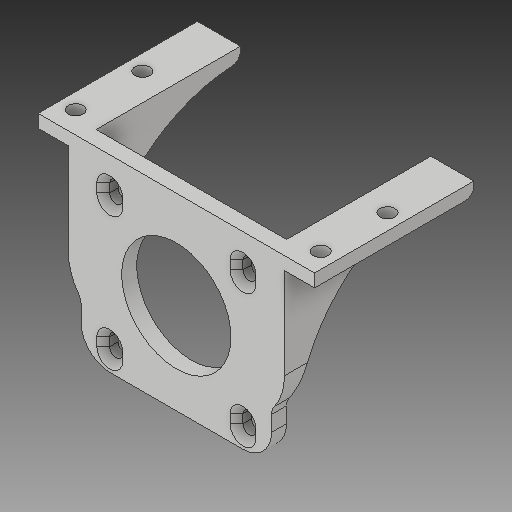
# Autodesk Inventor part: stepper mount
Saved by Autodesk Inventor 2017 (Build 210142000, 142)
## iProperties
Created: 2018-11-26
Part Number: stepper mount
Material: Generic
Document SubType Name: Modeling
Designer: Eric the Great
Density: 1 g/cm^3
Appearance: Default
Author: Eric the Great
Autodesk Inventor part; units mm, degrees
ref_plane "YZ Plane" through (0, 0, 0) normal (1, 0, 0) x (0, 1, 0)
ref_plane "XZ Plane" through (0, 0, 0) normal (0, 1, 0) x (-1, 0, 0)
ref_plane "XY Plane" through (0, 0, 0) normal (0, 0, 1) x (1, 0, 0)
sketch "Sketch1" plane through (0, 0, 0) normal (0, 0, 1) x (1, 0, 0)
  circle A0 centre (-15.5, -15.5) radius 1.5 projected
  circle A1 centre (15.5, 15.5) radius 1.5 projected
  circle A2 centre (15.5, -15.5) radius 1.5 projected
  circle A3 centre (-15.5, 15.5) radius 1.5 projected
  line L0 (21.15, 15.4142) -> (15.4142, 21.15) projected
  line L1 (15.4142, 21.15) -> (-15.4142, 21.15) projected
  line L2 (-21.15, 15.4142) -> (-15.4142, 21.15) projected
  line L3 (-21.15, 15.4142) -> (-21.15, -15.4142) projected
  line L4 (-21.15, -15.4142) -> (-15.4142, -21.15) projected
  line L5 (-15.4142, -21.15) -> (15.4142, -21.15) projected
  line L6 (21.15, -15.4142) -> (15.4142, -21.15) projected
  line L7 (21.15, -15.4142) -> (21.15, 15.4142) projected
  circle A4 centre (0, 0) radius 11 projected
  line L8 (22.15, 22.6799) -> (22.15, -14.4142)
  line L9 (15.4142, -21.15) -> (22.15, -14.4142)
  line L10 (-22.15, 22.6799) -> (-22.15, -14.4142)
  line L11 (-22.15, -14.4142) -> (-15.4142, -21.15)
  line L12 (0, 0) -> (0, -1.5411)
  line L13 (25, 22.6799) -> (-25, 22.6799) projected
  circle A5 centre (0, 0) radius 12.7
  arc A6 (15.4142, -21.15) -> (22.15, -14.4142) centre (15.4142, -14.4142) ccw
  arc A7 (-22.15, -14.4142) -> (-15.4142, -21.15) centre (-15.4142, -14.4142) ccw
  point P0 (0, 0)
  point P1 (0, 17)
  point P2 (22.15, 21.15)
  point P3 (-22.15, 21.15)
  dimension "d4" = 1
  dimension "d24" = 25.4
  constraints: 10 end point, 7 point on line, 4 point on circle, 4 tangent, 3 centre point, 2 collinear, 2 vertical, 1 coincident, 1 parallel, 1 other
  measures "d4" distance between parallel lines of L7 L8
  measures "d24" diameter of A5
extrude "Extrusion1" add sketch "Sketch1" along normal blind 3.5 contours L7 L6 L5 L4 L3 L2 L1 L0 | L0 L1 L2 L3 L11 L10 L13 L8 L9 L7 | L9 A6 L6 | A7 L11 L4
sketch "Sketch3" plane through (-22.15, -14.4142, 0) normal (-1, 0, 0) x (0, 0, 1)
  line L0 (-80.2095, 37.0941) -> (300.7905, 37.0941) projected
  line L1 (3.5, 37.0941) -> (3.5, 0) projected
  line L2 (3.5, 6.7772) -> (3.5, 37.0941)
  line L3 (-33.5642, 37.0941) -> (3.5, 37.0941)
  line L4 (0, 37.0941) -> (0, 0) projected
  arc A0 (0, 6.7772) -> (-32.2994, 34.0941) centre (-33.4606, -0.0326) ccw
  line L5 (-33.5642, 37.0941) -> (-33.5642, 34.0941)
  line L6 (-33.5642, 34.0941) -> (-32.2994, 34.0941)
  line L7 (3.5, 6.7772) -> (0, 6.7772)
  line L8 (-33.5642, 37.0941) -> (3.5, 37.0941)
  line L9 (3.5, 37.0941) -> (3.5, 33.5312)
  line L10 (-33.5642, 37.0941) -> (3.5, 37.0941)
  line L11 (3.5, 37.0941) -> (3.5, 33.5312)
  point P0 (0, 14.4142)
  point P1 (3, 35.5642)
  point P2 (0, 35.5642)
  dimension "d14" = 3
  constraints: 18 end point, 4 perpendicular, 4 point on line, 2 horizontal, 2 point on circle, 1 centre point, 1 collinear, 1 parallel, 1 vertical, 2 other
  measures "d14" distance of L3.start L5.end
extrude "Extrusion3" add sketch "Sketch3" along normal blind 3
sketch "Sketch4" plane through (22.15, -14.4142, 0) normal (1, 0, 0) x (0, 0, -1)
  arc A0 (32.2994, 34.0941) -> (0, 6.7772) centre (33.4606, -0.0326) ccw projected
  line L0 (33.5642, 34.0941) -> (32.2994, 34.0941) projected
  line L1 (33.5642, 37.0941) -> (33.5642, 34.0941) projected
  line L2 (-3.5, 6.7772) -> (0, 6.7772) projected
  line L3 (-3, 35.5642) -> (-3, 37.0941) projected
  line L4 (0, 37.0941) -> (0, 6.7772) projected
  arc A1 (32.2994, 34.0941) -> (0, 6.7772) centre (33.4606, -0.0326) ccw projected
  line L5 (33.5642, 34.0941) -> (32.2994, 34.0941) projected
  line L6 (33.5642, 37.0941) -> (33.5642, 34.0941) projected
  line L7 (0, 37.0941) -> (33.5642, 37.0941) projected
  line L8 (-3.5, 0) -> (-3.5, 37.0941) projected
  line L9 (0, 6.7772) -> (-3.5, 6.7772)
  line L10 (-3.5, 6.7772) -> (-3.5, 37.0941)
  line L11 (0, 6.7772) -> (-3.5, 6.7772)
  line L12 (-3.5, 6.7772) -> (-3.5, 37.0941)
  line L13 (-3.5, 37.0941) -> (0, 37.0941)
  line L14 (0, 37.0941) -> (0, 6.7772)
  point P0 (0, 14.4142)
  constraints: 12 end point, 2 parallel, 1 collinear, 1 horizontal, 1 perpendicular, 1 vertical, 1 other
extrude "Extrusion4" add sketch "Sketch4" along normal blind 3
sketch "Sketch5" plane through (-25.15, -14.4142, 0) normal (-1, 0, 0) x (0, 0, 1)
  line L0 (-33.5642, 37.0941) -> (3.5, 37.0941) projected
  line L1 (3.5, 37.0941) -> (3.5, 6.7772) projected
  line L2 (-33.5642, 37.0941) -> (3.5, 37.0941)
  line L3 (3.5, 37.0941) -> (3.5, 34.0941)
  line L4 (3.5, 34.0941) -> (-33.5642, 34.0941)
  line L5 (-33.5642, 34.0941) -> (-33.5642, 37.0941)
  point P0 (0, 14.4142)
  dimension "d9" = 3
  constraints: 8 end point, 2 parallel, 1 horizontal, 1 perpendicular, 1 point on line
  measures "d9" distance of L4.end L0.start
extrude "Extrusion5" add sketch "Sketch5" along normal blind 7
fillet "Fillet1" radius 3.175 2 edges at (-22.15, -7.6371, 1.75) (22.15, -7.6371, 1.75)
fillet "Fillet2" radius 12.7 4 edges at (25.15, -7.6395, 0) (25.15, -7.6419, 1.75) (-25.15, -7.6395, 0) (-25.15, -7.6419, 1.75)
sketch "Sketch6" plane through (25.15, -14.4142, 0) normal (1, 0, 0) x (0, 0, -1)
  line L0 (33.5642, 37.0941) -> (33.5642, 34.0941) projected
  line L1 (33.5642, 37.0941) -> (-3.5, 37.0941)
  line L2 (-3.5, 37.0941) -> (-3.5, 34.0941)
  line L3 (-3.5, 34.0941) -> (33.5642, 34.0941)
  line L4 (33.5642, 34.0941) -> (33.5642, 37.0941)
  line L5 (-3.5, 37.0941) -> (-3.5, 12.8941) projected
  point P0 (0, 14.4142)
  dimension "d15" = 3
  constraints: 8 end point, 2 parallel, 1 horizontal, 1 perpendicular, 1 point on line
  measures "d15" distance of L0.start L0.end
extrude "Extrusion6" add sketch "Sketch6" along normal blind 7
sketch "Sketch7" plane through (22.15, 19.6799, -33.5642) normal (0, -1, 0) x (1, 0, 0)
  circle A0 centre (6.35, 15.9631) radius 1.75 projected
  circle A1 centre (-50.65, 15.9631) radius 1.75 projected
  circle A2 centre (6.35, 31.9823) radius 1.75
  circle A3 centre (-50.65, 31.9823) radius 1.75
  circle A4 centre (6.35, 16.4631) radius 1.75 projected
  circle A5 centre (-50.65, 16.4631) radius 1.75 projected
  point P0 (-22.15, 33.5642)
  dimension "d18" = 3.5
  dimension "d19" = 3.5
  constraints: 2 centre point
  measures "d18" diameter of A2
  measures "d19" diameter of A3
extrude "Extrusion7" cut sketch "Sketch7" against normal up to surface (3 mm away) contours A4 A0 | A0 A4 | A5 A1 | A1 A5 | A2 | A3 picked at (6.4875, 16.6967) picked at (6.5821, 17.8556) picked at (-50.7875, 16.6967) picked at (-50.4179, 17.8556)
fillet "Fillet3" radius 2 2 edges at (27.15, 19.6799, -33.5642) (-27.15, 19.6799, -33.5642)
fillet "Fillet4" radius 2 2 edges at (23.65, 19.6995, -33.5642) (-23.65, 19.6995, -33.5642)
sketch "Sketch8" plane through (0, 0, 3.5) normal (0, 0, 1) x (1, 0, 0)
  arc A0 (-25.15, -1.5201) -> (-22.75, -8.9498) centre (-12.45, -1.5201) ccw projected
  arc A1 (-22.15, -10.8072) -> (-22.75, -8.9498) centre (-25.325, -10.8072) ccw projected
  line L0 (-22.15, -10.8072) -> (-22.15, -14.4142) projected
  line L1 (-15.4142, -21.15) -> (15.4142, -21.15) projected
  line L2 (22.15, -14.4142) -> (22.15, -10.8072) projected
  arc A2 (22.75, -8.9498) -> (22.15, -10.8072) centre (25.325, -10.8072) ccw projected
  arc A3 (22.75, -8.9498) -> (25.15, -1.5201) centre (12.45, -1.5201) ccw projected
  line L3 (25.15, 19.6799) -> (25.15, -1.5201) projected
  line L4 (25.15, 19.6799) -> (32.15, 19.6799) projected
  line L5 (32.15, 22.6799) -> (32.15, 19.6799) projected
  line L6 (-32.15, 22.6799) -> (32.15, 22.6799) projected
  line L7 (-32.15, 19.6799) -> (-32.15, 22.6799) projected
  line L8 (-25.15, 19.6799) -> (-32.15, 19.6799) projected
  line L9 (-25.15, -1.5201) -> (-25.15, 19.6799) projected
  circle A4 centre (-15.5, -15.5) radius 1.5 projected
  circle A5 centre (15.5, 15.5) radius 1.5 projected
  circle A6 centre (15.5, -15.5) radius 1.5 projected
  circle A7 centre (-15.5, 15.5) radius 1.5 projected
  circle A8 centre (0, 0) radius 12.7 projected
  line L10 (-15.5, 15.5) -> (-15.5, 13.5) construction
  line L11 (-17, 15.5) -> (-17, 13.5)
  line L12 (-14, 13.5) -> (-14, 15.5)
  arc A9 (-14, 15.5) -> (-17, 15.5) centre (-15.5, 15.5) ccw
  arc A10 (-17, 13.5) -> (-14, 13.5) centre (-15.5, 13.5) ccw
  line L13 (15.5, 15.5) -> (15.5, 13.5) construction
  line L14 (14, 15.5) -> (14, 13.5)
  line L15 (17, 13.5) -> (17, 15.5)
  arc A11 (17, 15.5) -> (14, 15.5) centre (15.5, 15.5) ccw
  arc A12 (14, 13.5) -> (17, 13.5) centre (15.5, 13.5) ccw
  line L16 (-15.5, -15.5) -> (-15.5, -17.5) construction
  line L17 (-14, -15.5) -> (-14, -17.5)
  line L18 (-17, -17.5) -> (-17, -15.5)
  arc A13 (-14, -15.5) -> (-17, -15.5) centre (-15.5, -15.5) ccw
  arc A14 (-17, -17.5) -> (-14, -17.5) centre (-15.5, -17.5) ccw
  circle A15 centre (15.5, -15.5) radius 1.5 projected
  line L19 (15.5, -15.5) -> (15.5, -17.5) construction
  line L20 (14, -15.5) -> (14, -17.5)
  line L21 (17, -17.5) -> (17, -15.5)
  arc A16 (17, -15.5) -> (14, -15.5) centre (15.5, -15.5) ccw
  arc A17 (14, -17.5) -> (17, -17.5) centre (15.5, -17.5) ccw
  arc A18 (-22.15, -14.4142) -> (-15.4142, -21.15) centre (-15.4142, -14.4142) ccw projected
  arc A19 (15.4142, -21.15) -> (22.15, -14.4142) centre (15.4142, -14.4142) ccw projected
  circle A20 centre (-15.5, -15.5) radius 1.5 projected
  point P0 (0, 0)
  point P1 (-15.5, 14.5)
  point P2 (15.5, 14.5)
  point P3 (-15.5, -16.5)
  point P4 (15.5, -16.5)
  dimension "d25" = 2
  constraints: 32 end point, 17 tangent, 16 point on circle, 8 centre point, 5 parallel, 4 midpoint, 3 equal length, 2 point on line, 1 vertical
  measures "d25" distance of L10.start L10.end
extrude "Extrusion8" cut sketch "Sketch8" against normal blind 25.4 contours A4 | L17 A14 L18 A4 | L15 A12 L14 A5 | L21 A17 L20 A6 | L12 A10 L11 A7
chamfer "Chamfer1" distance 1.5 angle 45 16 edges at (-15.5, -19, 3.5) (-17, -16.5, 3.5) (-15.5, -14, 3.5) (-14, -16.5, 3.5) (15.5, -19, 3.5) (14, -16.5, 3.5) (15.5, -14, 3.5) (17, -16.5, 3.5) (15.5, 12, 3.5) (14, 14.5, 3.5) (15.5, 17, 3.5) (17, 14.5, 3.5) (-15.5, 12, 3.5) (-17, 14.5, 3.5) (-15.5, 17, 3.5) (-14, 14.5, 3.5)
body "Solid1"
